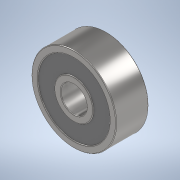
# Autodesk Inventor part: 624 Bearing
Saved by Autodesk Inventor 2020 (Build 240168000, 168)
## iProperties
Created: 2023-06-16
Part Number: 624 Bearing
Material: Steel, Carbon
Document SubType Name: Modeling
Designer: Ishaan
Density: 7.85 g/cm^3
Appearance: Semi-Polished
Author: Ishaan
Autodesk Inventor part; units mm, degrees
ref_plane "YZ Plane" through (0, 0, 0) normal (1, 0, 0) x (0, 1, 0)
ref_plane "XZ Plane" through (0, 0, 0) normal (0, 1, 0) x (-1, 0, 0)
ref_plane "XY Plane" through (0, 0, 0) normal (0, 0, 1) x (1, 0, 0)
sketch "Sketch1" plane through (0, 0, 0) normal (0, 0, 1) x (1, 0, 0)
  circle A0 centre (0, 0) radius 2
  circle A1 centre (0, 0) radius 6.5
  circle A2 centre (0, 0) radius 5.5
  circle A3 centre (0, 0) radius 3
  dimension "d0" = 4
  dimension "d1" = 13
  dimension "d2" = 1
  dimension "d3" = 1
  constraints: 4 centre point, 2 coincident
  measures "d0" diameter of A0
  measures "d1" diameter of A1
  measures "d2" radial gap between concentric circles of A1 A2
  measures "d3" radial gap between concentric circles of A0 A3
extrude "Extrusion1" add sketch "Sketch1" along normal mid plane 5
extrude "Extrusion2" add sketch "Sketch1" along normal mid plane 4.8 contours A2
fillet "Fillet1" radius 0.1 8 edges at (-6.5, 0, 2.5) (-6.5, 0, -2.5) (-2, 0, 2.5) (-5.5, 0, 2.5) (-3, 0, 2.5) (-2, 0, -2.5) (-3, 0, -2.5) (-5.5, 0, -2.5)
body "Solid1"
